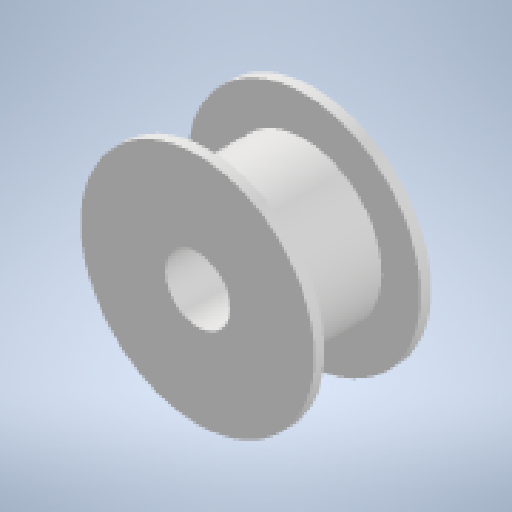
# Autodesk Inventor part: belt_gear_2
Saved by Autodesk Inventor 2024 (Build 280153000, 153)
## iProperties
Created: 2026-02-05
Part Number: belt_gear_2
Material: Generic
Document SubType Name: Modeling
Designer: SEMEN
Density: 1 g/cm^3
Appearance: Default
Author: SEMEN
Autodesk Inventor part; units mm, degrees
ref_plane "YZ Plane" through (0, 0, 0) normal (1, 0, 0) x (0, 1, 0)
ref_plane "XZ Plane" through (0, 0, 0) normal (0, 1, 0) x (-1, 0, 0)
ref_plane "XY Plane" through (0, 0, 0) normal (0, 0, 1) x (1, 0, 0)
sketch "Sketch1" plane through (0, 0, 0) normal (1, 0, 0) x (0, 1, 0)
  line L0 (0, 0) -> (9, 0)
  line L1 (9, 0) -> (9, 9)
  line L2 (9, 9) -> (0, 9)
  line L3 (0, 9) -> (0, 0)
  line L4 (9, 8.2) -> (2.5, 8.2)
  line L5 (9, 0.8) -> (2.5, 0.8)
  line L6 (6, 0.8) -> (6, 8.2)
  line L7 (2.5, 0) -> (2.5, 9)
  dimension "d0" = 9
  dimension "d1" = 9
  dimension "d2" = 7.4
  dimension "d3" = 0.8
  dimension "d4" = 2.5
  dimension "d5" = 6
  constraints: 16 end point, 8 point on line, 4 perpendicular, 2 horizontal, 2 parallel
  measures "d0" distance of L2.end L1.end
  measures "d1" distance of L1.end L0.end
  measures "d2" distance between parallel lines of L4 L5
  measures "d3" distance between parallel lines of L2 L4
  measures "d4" distance between parallel lines of L3 L7
  measures "d5" distance between parallel lines of L3 L6
revolve "Revolution1" add sketch "Sketch1" angle 360 about axis through (0, 0, 9) along (0, 0, -1) contours L7 L5 L1 L0 | L7 L4 L6 L5 | L2 L1 L4 L7
body "Solid1"
